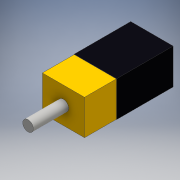
# Autodesk Inventor part: motor
Saved by Autodesk Inventor 2016 SP2 (Build 200236200, 236)
## iProperties
Created: 2017-02-02
Part Number: motor
Material: Generic
Document SubType Name: Modeling
Designer: Teta
Density: 1 g/cm^3
Appearance: Default
Author: Teta
Autodesk Inventor part; units mm, degrees
ref_plane "YZ Plane" through (0, 0, 0) normal (1, 0, 0) x (0, 1, 0)
ref_plane "XZ Plane" through (0, 0, 0) normal (0, 1, 0) x (-1, 0, 0)
ref_plane "XY Plane" through (0, 0, 0) normal (0, 0, 1) x (1, 0, 0)
sketch "Sketch1" plane through (0, 0, 0) normal (0, 1, 0) x (-1, 0, 0)
  circle A0 centre (0, 0) radius 1.5
  dimension "d0" = 3
  constraints: 1 centre point, 1 coincident
  measures "d0" diameter of A0
extrude "Extrusion1" add sketch "Sketch1" along normal blind 10
sketch "Sketch2" plane through (0, 10, 0) normal (0, 1, 0) x (1, 0, 0)
  line L0 (0, 0) -> (0, 4.95)
  line L1 (0, 4.95) -> (-5.95, 4.95)
  line L2 (-5.95, 4.95) -> (5.95, 4.95)
  line L3 (5.95, 4.95) -> (5.95, -4.95)
  line L4 (5.95, -4.95) -> (-5.95, -4.95)
  line L5 (-5.95, -4.95) -> (-5.95, 4.95)
  dimension "d3" = 4.95
  dimension "d4" = 5.95
  dimension "d5" = 11.9
  dimension "d6" = 9.9
  constraints: 12 end point, 2 parallel, 2 perpendicular, 1 horizontal, 1 vertical
  measures "d3" distance of L0.start L0.end
  measures "d4" distance of L0.end L1.end
  measures "d5" distance of L3.end L4.end
  measures "d6" distance of L2.end L3.end
extrude "Extrusion2" add sketch "Sketch2" along normal blind 9
sketch "Sketch3" plane through (0, 19, 0) normal (0, 1, 0) x (1, 0, 0)
  line L0 (0, 0) -> (6, 0)
  line L1 (6, 0) -> (6, 5)
  line L2 (6, 5) -> (-6, 5)
  line L3 (-6, 5) -> (-6, -5)
  line L4 (-6, -5) -> (6, -5)
  line L5 (6, -5) -> (6, 5)
  dimension "d9" = 6
  dimension "d10" = 5
  dimension "d11" = 12
  dimension "d12" = 10
  constraints: 12 end point, 2 horizontal, 2 parallel, 2 perpendicular
  measures "d9" distance of L0.start L0.end
  measures "d10" distance of L0.end L1.end
  measures "d11" distance of L4.end L3.end
  measures "d12" distance of L3.end L2.end
extrude "Extrusion3" add sketch "Sketch3" along normal blind 16
body "Solid1"
